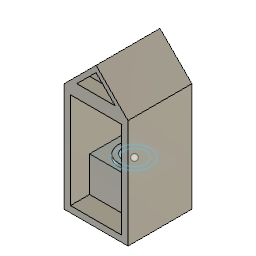
outHouse (Autodesk Fusion 360 design; units mm, degrees)
Autodesk Fusion 360 part; units mm, degrees
sketch "Sketch1" plane through (0, 0, 0) normal (0, 1, 0) x (1, 0, 0)
  line L0 (0, 0) -> (10, 0)
  line L1 (10, 0) -> (10, -17)
  line L2 (0, -17) -> (0, 0)
  line L3 (0, -17) -> (5, -22)
  line L4 (5, -22) -> (10, -17)
  dimension "d1" = 10
  dimension "d2" = 17
  constraint horizontal L0
  constraint vertical L1
  constraint vertical L2
  constraint coincident L0.start L2.end
  measures "d1" distance of L0.start L0.end
  measures "d2" distance of L0.start L2.start
extrude "Extrude1" add sketch "Sketch1" along normal blind 10
sketch "Sketch2" plane through (0, 0, 0) normal (0, 1, 0) x (1, 0, 0)
  line L0 (1, -1) -> (9, -1)
  line L1 (9, -1) -> (9, -16)
  line L2 (9, -16) -> (1, -16)
  line L3 (1, -16) -> (1, -1)
  line L4 (2, -18) -> (8, -18)
  line L5 (8, -18) -> (5, -21)
  line L6 (5, -21) -> (2, -18)
  constraint horizontal L0
  constraint vertical L1
  constraint horizontal L2
  constraint vertical L3
  constraint horizontal L4
extrude "Extrude2" cut sketch "Sketch2" along normal blind 2 contours L4 L5 L6
extrude "Extrude3" cut sketch "Sketch2" along normal blind 9 contours L0 L1 L2 L3
sketch "Sketch3" plane through (0, 9, 0) normal (0, -1, 0) x (1, 0, 0)
  line L0 (9, 16) -> (1, 16)
  line L1 (1, 16) -> (1, 1)
  line L2 (1, 1) -> (9, 1)
  line L3 (9, 1) -> (9, 16)
  line L4 (1, 1) -> (9, 1)
  line L5 (9, 1) -> (9, 6.5)
  line L6 (9, 6.5) -> (1, 6.5)
  line L7 (1, 6.5) -> (1, 1)
  constraint horizontal L4
  constraint vertical L5
  constraint horizontal L6
  constraint vertical L7
  constraint coincident L3 L5.end
  constraint coincident L1.end L2.start
extrude "Extrude4" add sketch "Sketch3" along normal blind 6 contours L1 L2 L3 L4 L5 L6 L7
sketch "Sketch4" plane through (0, 0, 6.5) normal (0, 0, 1) x (-1, 0, 0)
  line L0 (-9, -9) -> (-1, -9)
  line L1 (-1, -9) -> (-1, -3)
  line L2 (-1, -3) -> (-9, -3)
  line L3 (-9, -3) -> (-9, -9)
  circle A0 centre (-5, -6) radius 2.5
  circle A1 centre (-5, -6) radius 1.75
  dimension "d11" = 5
  dimension "d12" = 3.5
  constraint concentric A0 A1
  measures "d11" diameter of A0
  measures "d12" diameter of A1
extrude "Extrude5" add sketch "Sketch4" along normal blind 0.5 contours A0
extrude "Extrude6" cut sketch "Sketch4" against normal blind 3 contours A1
